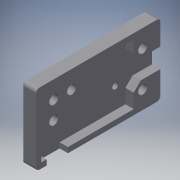
# Autodesk Inventor part: bumper cover lower
Saved by Autodesk Inventor 2019 (Build 230136000, 136)
## iProperties
Created: 2018-12-04
Part Number: bumper cover lower
Material: Generic
Document SubType Name: Modeling
Designer: Varga Daniel
Density: 1 g/cm^3
Appearance: Default
Author: Varga Daniel
Autodesk Inventor part; units mm, degrees
ref_plane "YZ Plane" through (0, 0, 0) normal (1, 0, 0) x (0, 1, 0)
ref_plane "XZ Plane" through (0, 0, 0) normal (0, 1, 0) x (-1, 0, 0)
ref_plane "XY Plane" through (0, 0, 0) normal (0, 0, 1) x (1, 0, 0)
sketch "Sketch1" plane through (0, 0, 0) normal (1, 0, 0) x (0, 1, 0)
  line L0 (-1.75, 0) -> (1.75, 0) construction
  arc A0 (2.75, -1) -> (1.75, 0) centre (1.75, -1) ccw construction
  line L1 (2.75, -1) -> (2.75, -4.5) construction
  line L2 (2.75, -4.5) -> (-0.75, -4.5) construction
  arc A1 (-1.75, -3.5) -> (-0.75, -4.5) centre (-0.75, -3.5) ccw construction
  line L3 (-1.75, -3.5) -> (-1.75, 0) construction
  circle A2 centre (0.5, -2.25) radius 1.55 construction
  line L4 (13.05, 17.7) -> (9.55, 17.7) construction
  arc A3 (8.55, 18.7) -> (9.55, 17.7) centre (9.55, 18.7) ccw construction
  line L5 (8.55, 18.7) -> (8.55, 22.2) construction
  line L6 (8.55, 22.2) -> (12.05, 22.2) construction
  arc A4 (13.05, 21.2) -> (12.05, 22.2) centre (12.05, 21.2) ccw construction
  line L7 (13.05, 21.2) -> (13.05, 17.7) construction
  line L8 (12.35, 19.85) -> (12.35, 20.05) construction
  arc A5 (12.35, 20.05) -> (9.25, 20.05) centre (10.8, 20.05) ccw construction
  line L9 (9.25, 20.05) -> (9.25, 19.85) construction
  arc A6 (9.25, 19.85) -> (12.35, 19.85) centre (10.8, 19.85) ccw construction
  circle A7 centre (10.8, 20.05) radius 1.65
  circle A8 centre (0.5, -2.25) radius 1.65
  line L10 (-14.2, 47.05) -> (25.8, 47.05)
  line L11 (25.8, 47.05) -> (25.8, -22.95)
  line L12 (25.8, -22.95) -> (-14.2, -22.95)
  line L13 (-14.2, -22.95) -> (-14.2, 47.05)
  circle A9 centre (15.8, 37.05) radius 4
  circle A10 centre (5.8, 37.05) radius 4
  circle A11 centre (15.8, 27.05) radius 4
  circle A12 centre (15.8, -12.95) radius 4
  circle A13 centre (-4.2, -12.95) radius 4
  point P0 (0, 0)
  dimension "d0" = 3.3
  dimension "d1" = 3.3
  dimension "d2" = 70
  dimension "d3" = 27
  dimension "d4" = 40
  dimension "d5" = 15
  dimension "d6" = 8
  dimension "d7" = 10
  dimension "d10" = 10
  dimension "d15" = 10
  dimension "d18" = 10
  dimension "d23" = 8
  dimension "d24" = 10
  dimension "d25" = 10
  dimension "d28" = 20
  constraints: 8 end point, 7 centre point, 3 horizontal, 2 coincident, 2 parallel, 1 perpendicular, 1 vertical, 6 other
  measures "d0" diameter of A7
  measures "d1" diameter of A8
  measures "d2" distance between parallel lines of L12 L10
  measures "d3" distance from line of A5.centre L10
  measures "d4" distance between parallel lines of L13 L11
  measures "d5" distance from line of A6.centre L11
  measures "d6" diameter of A9
  measures "d7" distance from line of A9.centre L11
  measures "d10" distance of A9.centre A10.centre
  measures "d15" distance from line of A9.centre L10
  measures "d18" distance of A9.centre A11.centre
  measures "d23" diameter of A12
  measures "d24" distance from line of A12.centre L12
  measures "d25" distance from line of A12.centre L11
  measures "d28" distance of A12.centre A13.centre
extrude "Extrusion1" add sketch "Sketch1" against normal blind 4.5 contours L10 L11 L12 L13 | A9 | A10 | A11 | A12 | A13
sketch "Sketch2" plane through (-4.5, 0, 0) normal (-1, 0, 0) x (0, 0, 1)
  circle A0 centre (-2.25, 0.5) radius 1.65 construction
  circle A1 centre (20.05, 10.8) radius 1.65 construction
  line L0 (47.05, -14.2) -> (47.05, 25.8) construction
  line L1 (47.05, 25.8) -> (-22.95, 25.8) construction
  line L2 (-22.95, 25.8) -> (-22.95, -14.2) construction
  line L3 (-22.95, -14.2) -> (47.05, -14.2) construction
  circle A2 centre (20.05, 10.8) radius 3.5
  circle A3 centre (-2.25, 0.5) radius 3.5
  point P0 (0, 0)
  dimension "d35" = 7
  dimension "d36" = 7
  constraints: 2 centre point, 2 coincident
  measures "d35" diameter of A2
  measures "d36" diameter of A3
extrude "Extrusion2" cut sketch "Sketch2" against normal blind 3
sketch "Sketch3" plane through (0, 0, 0) normal (1, 0, 0) x (0, 0, -1)
  circle A0 centre (2.25, 0.5) radius 1.65 projected
  circle A1 centre (-20.05, 10.8) radius 1.65 projected
  line L0 (-47.05, -14.2) -> (-47.05, 25.8) projected
  line L1 (22.95, -14.2) -> (-47.05, -14.2) projected
  line L2 (22.95, 25.8) -> (22.95, -14.2) projected
  line L3 (-47.05, 25.8) -> (22.95, 25.8) projected
  line L4 (19.95, 22.8) -> (19.95, -11.2)
  line L5 (19.95, -11.2) -> (-44.05, -11.2)
  line L6 (-44.05, -11.2) -> (-44.05, 22.8)
  line L7 (-44.05, 22.8) -> (19.95, 22.8)
  line L8 (-44.05, -1.2) -> (-29.05, -1.2)
  line L9 (-29.05, -1.2) -> (-29.05, 9.8)
  line L10 (-29.05, 9.8) -> (-23.05, 9.8)
  line L11 (-23.05, 9.8) -> (-23.05, 22.8)
  line L12 (7.95, -11.2) -> (7.95, 0.8)
  line L13 (7.95, 0.8) -> (19.95, 0.8)
  line L14 (19.95, 11.8) -> (7.95, 11.8)
  line L15 (7.95, 11.8) -> (7.95, 22.8)
  point P0 (0, 0)
  dimension "d39" = 3
  dimension "d42" = 13
  dimension "d43" = 21
  dimension "d44" = 24
  dimension "d45" = 15
  dimension "d46" = 12
  dimension "d47" = 11
  dimension "d48" = 12
  constraints: 24 end point, 6 point on line, 5 perpendicular, 2 horizontal, 1 collinear, 1 vertical, 3 other
  measures "d39" distance between parallel lines of L3 L7
  measures "d42" distance between parallel lines of L7 L10
  measures "d43" distance between parallel lines of L11 L6
  measures "d44" distance between parallel lines of L8 L7
  measures "d45" distance between parallel lines of L9 L6
  measures "d46" distance between parallel lines of L4 L12
  measures "d47" distance between parallel lines of L7 L14
  measures "d48" distance between parallel lines of L13 L5
extrude "Extrusion4" add sketch "Sketch3" along normal blind 4.7 contours L0 L3 L2 L1 | L4 L14 L15 L7 | L4 L5 L12 L13 | L11 L10 L9 L8 L6 L7
sketch "Sketch5" plane through (-4.5, 0, 0) normal (-1, 0, 0) x (0, 0, 1)
  circle A0 centre (20.05, 10.8) radius 3.5 construction
  circle A1 centre (-2.25, 0.5) radius 3.5 construction
  line L0 (47.05, -14.2) -> (47.05, 25.8) construction
  line L1 (47.05, 25.8) -> (-22.95, 25.8) construction
  line L2 (-22.95, 25.8) -> (-22.95, -14.2) construction
  line L3 (-22.95, -14.2) -> (47.05, -14.2) construction
  circle A2 centre (-12.95, -4.2) radius 4
  circle A3 centre (-12.95, 15.8) radius 4
  circle A4 centre (37.05, 15.8) radius 4
  line L4 (-22.95, -14.2) -> (-22.95, 25.8) construction
  circle A5 centre (27.05, 15.8) radius 4
  circle A6 centre (37.05, 5.8) radius 4
  point P0 (0, 0)
  dimension "d51" = 8
  dimension "d52" = 8
  dimension "d53" = 8
  dimension "d54" = 10
  dimension "d55" = 10
  dimension "d56" = 10
  dimension "d57" = 10
  dimension "d58" = 10
  dimension "d59" = 10
  dimension "d62" = 10
  dimension "d69" = 10
  constraints: 5 centre point, 1 horizontal, 1 vertical, 4 other
  measures "d51" diameter of A2
  measures "d52" diameter of A3
  measures "d53" diameter of A4
  measures "d54" distance from line of A4.centre L1
  measures "d55" distance from line of A4.centre L0
  measures "d56" distance from line of A3.centre L1
  measures "d57" distance from line of A3.centre L4
  measures "d58" distance from line of A2.centre L2
  measures "d59" distance from line of A2.centre L3
  measures "d62" distance of A4.centre A5.centre
  measures "d69" distance of A4.centre A6.centre
extrude "Extrusion5" cut sketch "Sketch5" against normal blind 0.8
sketch "Sketch6" plane through (-4.5, 0, 0) normal (-1, 0, 0) x (0, 0, 1)
  circle A0 centre (27.05, 15.8) radius 4 construction
  circle A1 centre (-12.95, 15.8) radius 4 construction
  circle A2 centre (-12.95, -4.2) radius 4 construction
  circle A3 centre (37.05, 15.8) radius 4 construction
  circle A4 centre (37.05, 5.8) radius 4 construction
  circle A5 centre (20.05, 10.8) radius 3.5 construction
  circle A6 centre (-2.25, 0.5) radius 3.5 construction
  line L0 (47.05, -14.2) -> (47.05, 25.8) construction
  line L1 (47.05, 25.8) -> (-22.95, 25.8) construction
  line L2 (-22.95, 25.8) -> (-22.95, -14.2) construction
  line L3 (-22.95, -14.2) -> (47.05, -14.2) construction
  point P0 (0, 0)
hole "Hole1" at (-4.5, 15.8, -12.95) at (-4.5, -4.2, -12.95) at (-4.5, 15.8, 27.05) at (-4.5, 15.8, 37.05) at (-4.5, 5.8, 37.05) direction (1, 0, 0) diameter 5 end through all
chamfer "Chamfer1" distance 4 angle 45 4 edges at (2.35, -1.2, 29.05) (2.35, 9.8, 23.05) (2.35, 0.8, -7.95) (2.35, 11.8, -7.95)
sketch "Sketch8" plane through (4.7, 0, 0) normal (1, 0, 0) x (0, 0, -1)
  line L0 (11.95, 11.8) -> (7.95, 15.8) construction
  line L1 (11.95, 11.8) -> (19.95, 11.8) construction
  line L2 (19.95, 11.8) -> (19.95, 0.8) construction
  line L3 (19.95, 0.8) -> (11.95, 0.8) construction
  line L4 (7.95, -3.2) -> (11.95, 0.8) construction
  line L5 (7.95, -3.2) -> (7.95, -11.2) construction
  line L6 (7.95, -11.2) -> (-44.05, -11.2) construction
  line L7 (-44.05, -11.2) -> (-44.05, -1.2) construction
  line L8 (-44.05, -1.2) -> (-33.05, -1.2) construction
  line L9 (-29.05, 2.8) -> (-33.05, -1.2) construction
  line L10 (-29.05, 2.8) -> (-29.05, 9.8) construction
  line L11 (-29.05, 9.8) -> (-27.05, 9.8) construction
  line L12 (-23.05, 13.8) -> (-27.05, 9.8) construction
  line L13 (-23.05, 13.8) -> (-23.05, 22.8) construction
  line L14 (-23.05, 22.8) -> (7.95, 22.8) construction
  line L15 (7.95, 22.8) -> (7.95, 15.8) construction
  circle A0 centre (-37.05, 15.8) radius 2.5 construction
  circle A1 centre (12.95, -4.2) radius 2.5 construction
  circle A2 centre (12.95, 15.8) radius 2.5 construction
  circle A3 centre (-27.05, 15.8) radius 2.5 construction
  circle A4 centre (-37.05, 5.8) radius 2.5 construction
  line L16 (-47.05, 25.8) -> (-47.05, -14.2) construction
  line L17 (-47.05, -14.2) -> (22.95, -14.2) construction
  line L18 (22.95, -14.2) -> (22.95, 25.8) construction
  line L19 (22.95, 25.8) -> (-47.05, 25.8) construction
  line L20 (-29.05, -11.2) -> (-29.05, -14.2)
  line L21 (-29.05, -14.2) -> (-41.05, -14.2)
  line L22 (-41.05, -14.2) -> (-41.05, -11.2)
  line L23 (19.95, 11.8) -> (19.95, 0.8) projected
  line L24 (19.95, 0.8) -> (22.95, 0.8)
  line L25 (22.95, 0.8) -> (22.95, 11.8)
  line L26 (22.95, 11.8) -> (19.95, 11.8)
  line L27 (19.95, 11.8) -> (19.95, 0.8)
  line L28 (-41.05, -11.2) -> (-29.05, -11.2)
  line L29 (7.95, -11.2) -> (-44.05, -11.2) projected
  point P0 (0, 0)
  dimension "d89" = 3
  dimension "d90" = 15
  constraints: 16 end point, 3 collinear, 3 parallel, 3 point on line, 1 horizontal, 1 perpendicular
  measures "d89" distance between parallel lines of L22 L7
  measures "d90" distance between parallel lines of L20 L7
extrude "Extrusion7" cut sketch "Sketch8" against normal up to surface (4.7 mm away)
chamfer "Chamfer2" distance 2 angle 45 4 edges at (-4.5, -14.2, 12.05) (-4.5, 5.8, -22.95) (-4.5, 25.8, 12.05) (-4.5, 5.8, 47.05)
fillet "Fillet1" radius 2 4 edges at (1.1, 25.8, -22.95) (1.1, -14.2, -22.95) (1.1, -14.2, 47.05) (1.1, 25.8, 47.05)
equation "\"d36\" = d35"
body "Solid1"
